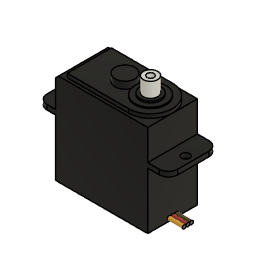
C6 (Autodesk Fusion 360 archive; units mm, degrees)
design "DS-R005 v3"
Autodesk Fusion 360 part; units mm, degrees
sketch "Sketch1" plane through (0, 0, 0) normal (0, 0, 1) x (1, 0, 0)
  circle A0 centre (0, 0) radius 2.35
  circle A1 centre (0, 0) radius 1.125
  dimension "d1" = 4.7
  dimension "d2" = 2.25
  constraint coincident A0.centre A1.centre
  constraint concentric A0 A1
  measures "d1" diameter of A0
  measures "d2" diameter of A1
extrude "Extrude1" add sketch "Sketch1" against normal blind 4.83 makes body 1
sketch "Sketch2" plane through (0, 0, -4.83) normal (0, 0, -1) x (1, 0, 0)
  circle A0 centre (0, 0) radius 1.125
  circle A1 centre (0, 0) radius 2.35
  circle A2 centre (0, 0) radius 3.38
  dimension "d5" = 6.76
  constraint concentric A0 A2
  measures "d5" diameter of A2
extrude "Extrude2" add sketch "Sketch2" along normal blind 0.54 contours A0 | A1 | A2 bodies 1
sketch "Sketch3" plane through (0, 0, -5.37) normal (0, 0, -1) x (1, 0, 0)
  circle A0 centre (0, 0) radius 3.38
  circle A1 centre (0, 0) radius 5.075
  dimension "d8" = 10.15
  constraint concentric A0 A1
  measures "d8" diameter of A1
extrude "Extrude3" add sketch "Sketch3" along normal blind 0.38 contours A0 | A1 bodies 1
sketch "Sketch4" plane through (0, 0, -5.75) normal (0, 0, -1) x (1, 0, 0)
  circle A0 centre (0, 0) radius 5.075
  circle A1 centre (0, 0) radius 7.165
  line L0 (0, 7.165) -> (-19.935, 7.165)
  line L1 (-19.935, 7.165) -> (-19.935, -7.165)
  line L2 (-19.935, -7.165) -> (0, -7.165)
  line L3 (0, -7.165) -> (0, 7.165)
  dimension "d11" = 14.33
  dimension "d12" = 19.935
  constraint coincident A0.centre A1.centre
  constraint horizontal L0
  constraint vertical L1
  constraint horizontal L2
  constraint vertical L3
  constraint coincident A1 L0.start
  constraint coincident A0.centre L3
  constraint tangent A1 L2
  measures "d11" diameter of A1
  measures "d12" distance of L1.end L2.end
extrude "Extrude4" add sketch "Sketch4" along normal blind 1.28 bodies 1
sketch "Sketch5" plane through (0, 0, -5.75) normal (0, 0, 1) x (-1, 0, 0)
  line L0 (0, -7.165) -> (19.935, -7.165)
  line L1 (19.935, -7.165) -> (19.935, 7.165)
  line L2 (19.935, 7.165) -> (0, 7.165)
  arc A0 (0, 7.165) -> (0, -7.165) centre (0, 0) ccw
  circle A1 centre (0, 0) radius 5.075
  circle A2 centre (8.31, 0) radius 3.235
  line L3 (19.935, 0) -> (-7.165, 0) construction
  dimension "d15" = 6.47
  constraint midpoint L1 L3.start
  constraint midpoint A0 L3.end
  constraint tangent A1 A2
  constraint coincident A2.centre L3
  measures "d15" diameter of A2
extrude "Extrude5" add sketch "Sketch5" along normal blind 2.27 separate body contours A2 makes body 2
sketch "Sketch6" plane through (0, 0, -7.03) normal (0, 0, -1) x (1, 0, 0)
  line L0 (-19.935, -7.165) -> (0, -7.165)
  arc A0 (0, -7.165) -> (0, 7.165) centre (0, 0) ccw
  line L1 (0, 7.165) -> (-19.935, 7.165)
  line L2 (-19.935, 7.165) -> (-19.935, -7.165)
  line L3 (7.165, 8.075) -> (-22.835, 8.075)
  line L4 (-22.835, 8.075) -> (-22.835, -8.075)
  line L5 (-22.835, -8.075) -> (7.165, -8.075)
  line L6 (7.165, -8.075) -> (7.165, 8.075)
  line L7 (0, -8.075) -> (0, 8.075) construction
  dimension "d18" = 30
  dimension "d21" = 16.15
  constraint horizontal L3
  constraint vertical L4
  constraint horizontal L5
  constraint vertical L6
  constraint tangent A0 L6
  constraint coincident L5 L7.start
  constraint coincident L3 L7.end
  constraint perpendicular L3 L7
  constraint midpoint A0.centre L7
  measures "d18" distance of L4.end L5.end
  measures "d21" distance of L3.start L5.end
extrude "Extrude6" add sketch "Sketch6" along normal blind 29.9 contours L0 A0 L1 L2 | L3 L4 L5 L6 bodies 1
chamfer "Chamfer1" distance 1 angle 45 1 edges at (-22.835, 0, -7.03) measured on face at (-22.835, -2.6917, -26.9633) on bodies 1
ref_plane "WorkPlane1" through (-7.335, 0, -16.93) normal (0, 0, 1) x (-1, 0, 0)
sketch "Sketch7" plane through (-7.335, 0, -16.93) normal (0, 0, 1) x (1, 0, 0)
  line L0 (21.25, -8.075) -> (-21.25, -8.075)
  line L1 (-21.25, -8.075) -> (-21.25, 8.075)
  line L2 (-21.25, 8.075) -> (21.25, 8.075)
  line L3 (21.25, 8.075) -> (21.25, -8.075)
  line L4 (21.25, -8.075) -> (-21.25, 8.075) construction
  line L5 (-21.25, -8.075) -> (21.25, 8.075) construction
  line L6 (-14.5, 8.075) -> (14.5, 8.075)
  circle A0 centre (18.8, 0) radius 1.3
  line L7 (0, 0) -> (0, -14.9185) construction
  line L8 (17.5, 2.3865) -> (17.5, -2.0248) construction
  line L9 (0, 0) -> (21.25, 0) construction
  circle A1 centre (-18.8, 0) radius 1.3
  dimension "d25" = 42.5
  dimension "d26" = 2.6
  dimension "d27" = 17.5
  constraint horizontal L0
  constraint perpendicular L0 L1
  constraint parallel L0 L2
  constraint parallel L1 L3
  constraint coincident L4 L7.start
  constraint coincident L5 L7.start
  constraint coincident L7.start L9.start
  constraint collinear L2 L6
  constraint perpendicular L0 L7
  constraint vertical L8
  constraint tangent A0 L8
  constraint midpoint L3 L9.end
  constraint coincident A0.centre L9
  constraint symmetric A0 L7 A1
  measures "d25" distance of L0.start L0.end
  measures "d26" diameter of A0
  measures "d27" distance of L7 L8
extrude "Extrude7" add sketch "Sketch7" against normal blind 1.58 bodies 1
sketch "Sketch8" plane through (-22.835, 0, 0) normal (-1, 0, 0) x (0, -1, 0)
  line L0 (8.075, -18.51) -> (-8.075, -18.51)
  line L1 (-8.075, -18.51) -> (-8.075, -36.93)
  line L2 (-8.075, -36.93) -> (8.075, -36.93)
  line L3 (8.075, -36.93) -> (8.075, -18.51)
  circle A0 centre (0, -35.95) radius 0.6
  circle A1 centre (1.2, -35.95) radius 0.6
  circle A2 centre (-1.2, -35.95) radius 0.6
  line L4 (1.2, -35.95) -> (-1.2, -35.95) construction
  line L5 (0, -35.95) -> (0, -36.93) construction
  dimension "d30" = 1.2
  dimension "d31" = 1.2
  dimension "d32" = 1.2
  dimension "d33" = 0.98
  constraint tangent A0 A2
  constraint tangent A0 A1
  constraint coincident A1.centre L4.start
  constraint parallel L2 L4
  constraint midpoint A0.centre L4
  constraint coincident A2.centre L4
  constraint coincident A0.centre L5.start
  constraint coincident L2 L5.end
  constraint perpendicular L2 L5
  constraint midpoint L2 L5.end
  measures "d30" diameter of A1
  measures "d31" diameter of A0
  measures "d32" diameter of A2
  measures "d33" distance of L2 A0.centre
extrude "Extrude8" add sketch "Sketch8" along normal blind 5 separate body contours A0 | A2 | A1 makes body 3
fillet "Fillet1" radius 3 4 edges at (-28.585, -8.075, -17.72) (-28.585, 8.075, -17.72) (13.915, -8.075, -17.72) (13.915, 8.075, -17.72) on bodies 1
move_body "Move1" bodies 3 to x (1, 0, 0) y (0, 1, 0) z (0, 0, 1) at (35, 0, 0)
equation "d12 = 27.1 mm - ( d11 / 2 )"
equation "d27 = ( 35 / 2 ) * 1 mm"
equation "d31 = d30"
equation "d32 = d31"
equation "d33 = 1.58 mm - 0.6 mm"
